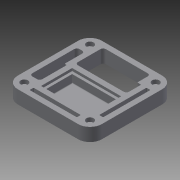
# Autodesk Inventor part: 14 pin short holder
Saved by Autodesk Inventor 2015 (Build 190159000, 159)
## iProperties
Created: 2014-12-11
Part Number: 14 pin short holder
Material: Generic
Document SubType Name: Modeling
Designer: Purple
Density: 1 g/cm^3
Appearance: Default
Author: Purple
Autodesk Inventor part; units mm, degrees
ref_plane "YZ Plane" through (0, 0, 0) normal (1, 0, 0) x (0, 1, 0)
ref_plane "XZ Plane" through (0, 0, 0) normal (0, 1, 0) x (-1, 0, 0)
sketch "Sketch1" plane through (0, 0, 0) normal (0, 1, 0) x (-1, 0, 0)
  line L0 (30, 30) -> (-30, 30)
  line L1 (-30, 30) -> (-30, -30)
  line L2 (-30, -30) -> (30, -30)
  line L3 (30, -30) -> (30, 30)
  line L4 (30, 30) -> (-30, -30) construction
  line L5 (-30, 30) -> (30, -30) construction
  point P0 (0, 0)
  dimension "d0" = 60
  dimension "d1" = 60
  constraints: 12 end point, 2 midpoint, 2 parallel, 1 horizontal, 1 perpendicular
  measures "d0" distance of L2.end L1.end
  measures "d1" distance of L0.end L1.end
extrude "Extrusion1" add sketch "Sketch1" along normal blind 10
fillet "Fillet1" radius 7 4 edges at (30, 5, 30) (30, 5, -30) (-30, 5, 30) (-30, 5, -30)
sketch "Sketch2" plane through (0, 10, 0) normal (0, 1, 0) x (1, 0, 0)
  line L0 (-30, 30) -> (30, 30)
  line L1 (30, 30) -> (30, -30)
  line L2 (30, -30) -> (-30, -30)
  line L3 (-30, -30) -> (-30, 30)
  line L4 (-30, 30) -> (30, -30) construction
  line L5 (30, 30) -> (-30, -30) construction
  line L6 (25, -25) -> (25, 25)
  line L7 (25, 25) -> (-25, 25)
  line L8 (-25, 25) -> (-25, -25)
  line L9 (-25, -25) -> (25, -25)
  circle A0 centre (25, -25) radius 2.75
  circle A1 centre (-25, -25) radius 2.75
  circle A2 centre (25, 25) radius 2.75
  circle A3 centre (-25, 25) radius 2.75
  point P0 (0, 0)
  dimension "d5" = 5
  dimension "d6" = 5.5
  dimension "d7" = 5.5
  dimension "d8" = 5.5
  dimension "d9" = 5.5
  constraints: 20 end point, 4 centre point, 4 coincident, 4 parallel, 2 midpoint, 2 perpendicular, 1 horizontal, 3 other
  measures "d5" distance between parallel lines of L1 L6
  measures "d6" diameter of A0
  measures "d7" diameter of A1
  measures "d8" diameter of A2
  measures "d9" diameter of A3
extrude "Extrusion2" cut sketch "Sketch2" against normal blind 3 contours L9 A0 L6 | L6 A0 L9 | A2 L7 L6 | L6 L7 A2 | A1 L8 L9 | L9 L8 A1 | A3 L8 L7 | L7 L8 A3
sketch "Sketch7" plane through (0, 10, 0) normal (0, 1, 0) x (1, 0, 0)
  line L0 (-23, 30) -> (23, 30)
  line L1 (30, 23) -> (30, -23)
  line L2 (23, -30) -> (-23, -30)
  line L3 (-30, -23) -> (-30, 23)
  line L4 (-30, 30) -> (30, -30) construction
  line L5 (30, 30) -> (-30, -30) construction
  arc A0 (-23, 30) -> (-30, 23) centre (-23, 23) ccw
  arc A1 (-30, -23) -> (-23, -30) centre (-23, -23) ccw
  arc A2 (23, -30) -> (30, -23) centre (23, -23) ccw
  arc A3 (30, 23) -> (23, 30) centre (23, 23) ccw
  line L6 (23, 32) -> (-23, 32)
  arc A4 (-23, 32) -> (-32, 23) centre (-23, 23) ccw
  line L7 (-32, 23) -> (-32, -23)
  arc A5 (-32, -23) -> (-23, -32) centre (-23, -23) ccw
  line L8 (-23, -32) -> (23, -32)
  arc A6 (23, -32) -> (32, -23) centre (23, -23) ccw
  line L9 (32, -23) -> (32, 23)
  arc A7 (32, 23) -> (23, 32) centre (23, 23) ccw
  point P0 (0, 0)
  dimension "d47" = 7
  dimension "d48" = 2
  constraints: 20 end point, 16 point on circle, 8 centre point, 8 point on line, 8 tangent, 4 parallel, 3 equal radius, 2 midpoint, 2 perpendicular, 1 horizontal, 7 other
  measures "d47" radius of A0
  measures "d48" distance between parallel lines of L0 L6
extrude "Extrusion6" add sketch "Sketch7" against normal blind 10
sketch "Sketch14" plane through (0, 10, 0) normal (0, 1, 0) x (1, 0, 0)
  line L0 (-25, 25) -> (25, 25)
  line L1 (25, 25) -> (25, -25)
  line L2 (25, -25) -> (-25, -25)
  line L3 (-25, -25) -> (-25, 25)
  line L4 (-25, 25) -> (25, -25) construction
  line L5 (25, 25) -> (-25, -25) construction
  line L6 (21, -21) -> (21, 2.7)
  line L7 (21, 21) -> (-21, 21)
  line L8 (-21, 21) -> (-21, -21)
  line L9 (-16.3, -21) -> (21, -21)
  line L10 (-16.3, -21) -> (-16.3, 2.7)
  line L11 (21, 2.7) -> (-16.3, 2.7)
  line L12 (19, 0.7) -> (-14.3, 0.7)
  line L13 (-14.3, 0.7) -> (-14.3, -19)
  line L14 (-19, -19) -> (-19, 19)
  line L15 (-19, 19) -> (19, 19)
  line L16 (19, -19) -> (-14.3, -19)
  line L17 (19, 0.7) -> (19, -19)
  point P0 (0, 0)
  dimension "d95" = 50
  dimension "d96" = 50
  dimension "d97" = 4
  dimension "d98" = 37.3
  dimension "d99" = 23.7
  dimension "d100" = 2
  constraints: 36 end point, 6 parallel, 6 perpendicular, 2 midpoint, 1 horizontal, 2 other
  measures "d95" distance of L1.end L2.end
  measures "d96" distance of L0.end L1.end
  measures "d97" distance between parallel lines of L1 L6
  measures "d98" distance of L9.start L6.start
  measures "d99" distance of L6.end L6.start
  measures "d100" distance between parallel lines of L11 L12
extrude "Extrusion12" cut sketch "Sketch14" against normal blind 2 contours L9 L10 L11 L6
sketch "Sketch15" plane through (0, 10, 0) normal (0, 1, 0) x (1, 0, 0)
  line L0 (-14.3, 0.7) -> (19, 0.7)
  line L1 (19, 0.7) -> (19, -19)
  line L2 (19, -19) -> (-14.3, -19)
  line L3 (-14.3, -19) -> (-14.3, 0.7)
  point P0 (0, 0)
  constraints: 8 end point, 2 parallel, 1 horizontal, 1 perpendicular
extrude "Extrusion13" cut sketch "Sketch15" against normal blind 8
sketch "Sketch16" plane through (0, 10, 0) normal (0, 1, 0) x (1, 0, 0)
  line L0 (23, 32) -> (-23, 32) projected
  line L1 (-32, 23) -> (-32, -23) projected
  line L2 (32, -23) -> (32, 23) projected
  line L3 (-18, 28) -> (18, 28)
  line L4 (-16.3, 2.7) -> (21, 2.7) projected
  line L5 (-18, 28) -> (-18, 6.7)
  line L6 (-18, 6.7) -> (18, 6.7)
  line L7 (18, 18) -> (18, 28)
  line L8 (-23, -32) -> (23, -32) projected
  line L9 (-16.3, -21) -> (-16.3, 2.7) projected
  line L10 (-28, -18) -> (-20.3, -18)
  line L11 (-20.3, -18) -> (-20.3, 2.7)
  line L12 (-28, -18) -> (-28, 18)
  line L13 (-20.3, 2.7) -> (-22, 2.7)
  line L14 (-22, 2.7) -> (-22, 6.7)
  line L15 (-28, 18) -> (-22, 18)
  line L16 (-22, 18) -> (-22, 6.7)
  line L17 (21, -21) -> (-16.3, -21) projected
  line L18 (18, -28) -> (18, -25)
  line L19 (18, -25) -> (-18, -25)
  line L20 (18, -28) -> (-18, -28)
  line L21 (-18, -28) -> (-18, -25)
  line L22 (21, 2.7) -> (21, -21) projected
  line L23 (28, 18) -> (28, -18)
  line L24 (28, -18) -> (25, -18)
  line L25 (25, -18) -> (25, 18)
  line L26 (28, 18) -> (25, 18)
  line L27 (21, 18) -> (21, 6.7)
  line L28 (21, 6.7) -> (18, 6.7)
  line L29 (21, 18) -> (18, 18)
  point P0 (0, 0)
  dimension "d106" = 4
  dimension "d107" = 4
  dimension "d108" = 14
  dimension "d109" = 14
  dimension "d110" = 4
  dimension "d111" = 4
  dimension "d112" = 4
  dimension "d113" = 14
  dimension "d114" = 4
  dimension "d115" = 14
  dimension "d116" = 4
  dimension "d117" = 4
  dimension "d118" = 4
  dimension "d119" = 4
  dimension "d120" = 4
  dimension "d121" = 14
  dimension "d122" = 4
  dimension "d123" = 14
  dimension "d124" = 4
  dimension "d125" = 14
  dimension "d126" = 4
  dimension "d127" = 4
  dimension "d128" = 14
  dimension "d129" = 4
  constraints: 44 end point, 9 perpendicular, 3 horizontal, 3 vertical, 1 collinear, 1 parallel
  measures "d106" distance from line of L3.start L0
  measures "d107" distance from line of L0 L3.end
  measures "d108" distance from line of L3.start L1
  measures "d109" distance from line of L3.end L2
  measures "d110" distance from line of L6.end L4
  measures "d111" distance from line of L4 L5.end
  measures "d112" distance from line of L1 L12.end
  measures "d113" distance from line of L12.end L0
  measures "d114" distance from line of L1 L10.start
  measures "d115" distance from line of L10.start L8
  measures "d116" distance from line of L9 L10.end
  measures "d117" vertical distance of L11.end L5.end
  measures "d118" distance of L5.end L14.end
  measures "d119" distance from line of L8 L18.start
  measures "d120" distance from line of L18.end L17
  measures "d121" distance from line of L18.start L2
  measures "d122" distance from line of L8 L20.end
  measures "d123" distance from line of L1 L20.end
  measures "d124" distance from line of L23.end L2
  measures "d125" distance from line of L23.end L8
  measures "d126" distance from line of L22 L24.end
  measures "d127" distance from line of L23.start L2
  measures "d128" distance from line of L0 L23.start
  measures "d129" distance from line of L25 L27.start
extrude "Extrusion14" cut sketch "Sketch16" against normal through all contours L3 L7 L29 L27 L28 L6 L5 | L12 L15 L16 L14 L13 L11 L10 | L20 L21 L19 L18 | L23 L24 L25 L26
fillet "Fillet4" radius 2 8 edges at (18, 5, -28) (-22, 5, -18) (-18, 5, -28) (-28, 5, -18) (-28, 5, 18) (-18, 5, -6.7) (-20.3, 5, 18) (21, 5, -6.7)
fillet "Fillet4" radius 0.5 16 edges at (28, 5, 18) (18, 5, 28) (28, 5, -18) (21, 5, -18) (18, 5, -18) (18, 5, 25) (-20.3, 5, -2.7) (-22, 5, -2.7) (25, 5, -18) (-18, 5, 25) (-18, 5, 28) (25, 5, 18) (-14.3, 2, 9.15) (2.35, 2, -0.7) (2.35, 2, 19) (19, 2, 9.15)
ref_plane "Work Plane3" through (0, 5, 0) normal (0, 1, 0) x (1, 0, 0)
mirror "Mirror3" about plane through (0, 5, 0) normal (0, 1, 0) of "Extrusion2"
body "Solid1"
